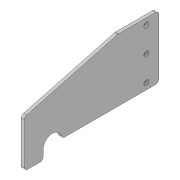
# Autodesk Inventor part: Handle_Bracket
Saved by Autodesk Inventor 2019.3 (Build 233278000, 278)
## iProperties
Created: 2019-01-15
Part Number: Handle_Bracket
Material: Generic
Document SubType Name: Modeling
Designer: Kathryn Rosie
Density: 1 g/cm^3
Appearance: Default
Author: Kathryn Rosie
Autodesk Inventor part; units mm, degrees
ref_plane "YZ Plane" through (0, 0, 0) normal (1, 0, 0) x (0, 1, 0)
ref_plane "XZ Plane" through (0, 0, 0) normal (0, 1, 0) x (-1, 0, 0)
ref_plane "XY Plane" through (0, 0, 0) normal (0, 0, 1) x (1, 0, 0)
sketch "Sketch1" plane through (0, 0, 0) normal (1, 0, 0) x (0, 1, 0)
  arc A0 (3.75, -14.5237) -> (0, 15) centre (0, 0) ccw
  line L0 (0, 45) -> (56.1586, 45)
  line L1 (100, -105.6552) -> (100, -150)
  line L2 (0, -150) -> (0, -19.3649)
  line L3 (0, 15) -> (-10, 15)
  line L4 (0, 15) -> (10, 15) construction
  line L5 (-15, 20) -> (-15, 40)
  line L6 (-10, 45) -> (0, 45)
  arc A1 (3.75, -14.5237) -> (0, -19.3649) centre (5, -19.3649) ccw
  arc A2 (-15, 20) -> (-10, 15) centre (-10, 20) ccw
  arc A3 (-10, 45) -> (-15, 40) centre (-10, 40) ccw
  line L7 (60.9898, 41.2883) -> (99.8312, -104.3669)
  line L8 (0, -150) -> (0, -165)
  line L9 (5, -170) -> (95, -170)
  line L10 (100, -165) -> (100, -150)
  circle A4 centre (90, -150) radius 4
  circle A5 centre (50, -150) radius 4
  circle A6 centre (10, -150) radius 4
  arc A7 (60.9898, 41.2883) -> (56.1586, 45) centre (56.1586, 40) ccw
  arc A8 (100, -105.6552) -> (99.8312, -104.3669) centre (95, -105.6552) ccw
  arc A9 (95, -170) -> (100, -165) centre (95, -165) ccw
  arc A10 (0, -165) -> (5, -170) centre (5, -165) ccw
  point P0 (60, 45)
  point P1 (-15, 15)
  point P2 (0, -15)
  point P3 (100, -105)
  point P4 (0, -170)
  point P5 (100, -170)
  dimension "d9" = 30
  dimension "d10" = 100
  dimension "d12" = 45
  dimension "d14" = 15
  dimension "d15" = 180
  dimension "d16" = 5
  dimension "d17" = 40
  dimension "d18" = 150
  dimension "d19" = 100
  dimension "d20" = 20
  dimension "d21" = 8
  dimension "d22" = 8
  dimension "d23" = 8
  dimension "d24" = 40
  dimension "d25" = 40
  dimension "d26" = 10
  dimension "d27" = 5
  dimension "d28" = 20
  dimension "d31" = 15
  dimension "d32" = 150
  constraints: 22 end point, 17 point on circle, 15 tangent, 11 centre point, 11 point on line, 5 equal radius, 4 horizontal, 2 collinear, 2 horizontal alignment, 2 parallel, 2 perpendicular, 1 coincident, 1 vertical
  measures "d9" diameter of A0
  measures "d10" distance of L2.start L1.end
  measures "d12" distance from line of L0 A0.centre
  measures "d14" distance of L3.start point (-15, 15)
  measures "d15" angle of L3 L4
  measures "d16" radius of A1
  measures "d17" distance from line of point (60, 45) L1
  measures "d18" distance from line of point (100, -105) L0
  measures "d19" distance of point (0, -170) point (100, -170)
  measures "d20" distance of point (100, -170) L1.end
  measures "d21" diameter of A4
  measures "d22" diameter of A5
  measures "d23" diameter of A6
  measures "d24" distance of A5.centre A4.centre
  measures "d25" distance of A6.centre A5.centre
  measures "d26" distance from line of L10 A4.centre
  measures "d27" radius of A7
  measures "d28" distance from line of L9 A4.centre
  measures "d31" distance between parallel lines of L5 L2
  measures "d32" vertical distance of A6.centre A0.centre
extrude "Extrusion1" add sketch "Sketch1" along normal blind 5
equation "\"d19\" = d10"
body "Solid1"
